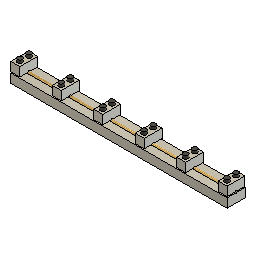
Shaft Cutting Jig (for cutting flats) (Autodesk Fusion 360 design; units mm, degrees)
Autodesk Fusion 360 part; units mm, degrees
note: some values were not read from the file. Chosen so that the rebuilt part matches the saved one: which bodies a step acts on.
sketch "Sketch1" plane through (0, 0, 0) normal (0, 1, 0) x (1, 0, 0)
  line L0 (0, 0) -> (304.8, 0)
  line L1 (304.8, 0) -> (304.8, -25.4)
  line L2 (304.8, -25.4) -> (0, -25.4)
  line L3 (0, -25.4) -> (0, 0)
  dimension "d1" = 304.8
  dimension "d2" = 25.4
  measures "d1" distance of L0.start L0.end
  measures "d2" distance of L0.start L2.end
extrude "Extrude1" add sketch "Sketch1" along normal blind 12.7 makes body 1
sketch "Sketch2" plane through (0, 0, 0) normal (-1, 0, 0) x (0, 0, 1)
  line L0 (0, 0) -> (25.4, 0)
  line L1 (25.4, 0) -> (25.4, 12.7)
  line L2 (25.4, 12.7) -> (0, 12.7)
  line L3 (0, 12.7) -> (0, 0)
  circle A0 centre (12.7, 13.462) radius 1.5875
  line L4 (0.2576, 14.224) -> (25.4, 14.224)
  line L5 (25.4, 14.224) -> (25.4, 26.924)
  line L6 (25.4, 26.924) -> (0.2576, 26.924)
  line L7 (0.2576, 26.924) -> (0.2576, 14.224)
  line L8 (10.4549, 13.462) -> (12.7, 11.2169)
  line L9 (12.7, 11.2169) -> (14.9451, 13.462)
  line L10 (14.9451, 13.462) -> (12.7, 15.7071)
  line L11 (12.7, 15.7071) -> (10.4549, 13.462)
  line L12 (12.7, 13.462) -> (12.7, 0) construction
  line L13 (10.4549, 13.462) -> (14.9451, 13.462) construction
  dimension "d5" = 3.175
  dimension "d6" = 0.762
  dimension "d7" = 12.7
  dimension "d8" = 0.762
  measures "d5" diameter of A0
  measures "d6" distance of L2 A0.centre
  measures "d7" distance of L4.end L5.end
  measures "d8" distance of A0.centre L4
extrude "Extrude2" add sketch "Sketch2" against normal blind 12.7 separate body contours A0 L4 | L4 L5 L6 L7 L10 L11 | A0 L10 L11 makes body 2
extrude "Extrude3" cut sketch "Sketch2" against normal through all contours L2 A0 L4 L8 L11 | L2 A0 L8 | L2 A0 L9 | L2 A0 L4 L9 L10 | L2 A0 L4 | L2 A0 | A0 L8 L9 | A0 L4 L11 | A0 L4 | A0 L4 L10 | A0 L10 L11 bodies 1 2
extrude "Extrude4" add sketch "Sketch2" against normal up to surface (304.8 mm away) separate body contours L2 A0 L4 | L2 A0 | A0 L4 makes body 3
sketch "Sketch3" plane through (0, 26.924, 0) normal (0, 1, 0) x (-1, 0, 0)
  line L0 (0, 0.2576) -> (0, 25.4)
  line L1 (0, 25.4) -> (-12.7, 25.4)
  line L2 (-12.7, 25.4) -> (-12.7, 0.2576)
  line L3 (-12.7, 0.2576) -> (0, 0.2576)
  line L4 (-6.35, 0.2576) -> (-6.35, 25.4) construction
  circle A0 centre (-6.35, 6.35) radius 2.25
  circle A1 centre (-6.35, 19.05) radius 2.25
  line L5 (0, 12.7) -> (-12.7, 12.7) construction
  point P0 (0, 12.7)
  point P1 (-12.7, 12.7)
  dimension "d14" = 4.5
  dimension "d15" = 4.5
  dimension "d16" = 6.35
  dimension "d17" = 6.35
  measures "d14" diameter of A0
  measures "d15" diameter of A1
  measures "d16" distance of A1.centre L5
  measures "d17" distance of A0.centre L5
extrude "Extrude5" cut sketch "Sketch3" against normal through all contours A0 | A1 bodies 1 2
sketch "Sketch4" plane through (0, 26.924, 0) normal (0, 1, 0) x (-1, 0, 0)
  circle A0 centre (-6.35, 19.05) radius 2.25
  circle A1 centre (-6.35, 6.35) radius 2.25
  line L0 (0, 0.2576) -> (0, 25.4)
  line L1 (0, 25.4) -> (-12.7, 25.4)
  line L2 (-12.7, 25.4) -> (-12.7, 0.2576)
  line L3 (-12.7, 0.2576) -> (0, 0.2576)
  circle A2 centre (-6.35, 6.35) radius 3.5
  circle A3 centre (-6.35, 19.05) radius 3.5
  dimension "d19" = 7
  dimension "d20" = 7
  measures "d19" diameter of A2
  measures "d20" diameter of A3
extrude "Extrude6" add sketch "Sketch4" along normal blind 4 separate body contours A0 | A1 | A2 | A3 makes body 4 at (2.8674, 28.2573, 18.7015) makes body 5 at (2.8674, 28.2573, 6.0015)
sketch "Sketch6" plane through (0, 26.924, 0) normal (0, -1, 0) x (1, 0, 0)
  circle A0 centre (6.35, 6.35) radius 3.5
  circle A1 centre (6.35, 19.05) radius 3.5
  circle A2 centre (6.35, 6.35) radius 2
  circle A3 centre (6.35, 19.05) radius 2
  dimension "d32" = 4
  dimension "d33" = 4
  measures "d32" diameter of A2
  measures "d33" diameter of A3
extrude "Extrude7" add sketch "Sketch6" along normal blind 25 contours A2 | A3 bodies 4 5
pattern_linear "R-Pattern1" count 6 spacing 58.42 along (1, 0, 0) of bodies 2 4 5 makes body 6 at (58.42, 23.185, 12.7859) makes body 7 at (116.84, 23.185, 12.7859) makes body 8 at (175.26, 23.185, 12.7859) makes body 9 at (233.68, 23.185, 12.7859) makes body 10 at (292.1, 23.185, 12.7859) makes body 11 at (66.7601, 18.5907, 18.8509) makes body 12 at (125.1801, 18.5907, 18.8509) makes body 13 at (182.7775, 10.2573, 20.6739) makes body 14 at (241.1975, 10.2573, 20.6739) makes body 15 at (300.293, 10.2573, 19.8269) makes body 16 at (66.0934, 10.2573, 7.8496) makes body 17 at (121.7935, 10.2573, 7.7817) makes body 18 at (180.6976, 18.5907, 4.5703) makes body 19 at (239.1176, 18.5907, 4.5703) makes body 20 at (299.3624, 10.2573, 8.1297)
pattern_linear "R-Pattern2" count 6 spacing 58.42 along (1, 0, 0) of "Extrude5"
equation "d8 = d6"
